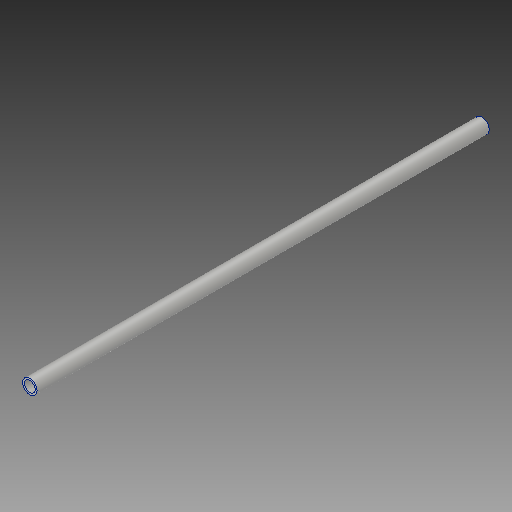
# Autodesk Inventor part: aluminium_bar_D8_L250
Saved by Autodesk Inventor 2019 (Build 230136000, 136)
## iProperties
Created: 2018-10-30
Part Number: aluminium_bar_D8_L250
Material: Aluminum 6061
Document SubType Name: Modeling
Designer: Gianpietro
Density: 2.7 g/cm^3
Appearance: Aluminum - Flat
Mass: 14.844 g
Surface Area: 110.396 cm^2
Volume: 5.49779 cm^3
Author: Gianpietro
Autodesk Inventor part; units mm, degrees
ref_plane "YZ Plane" through (0, 0, 0) normal (1, 0, 0) x (0, 1, 0)
ref_plane "XZ Plane" through (0, 0, 0) normal (0, 1, 0) x (-1, 0, 0)
ref_plane "XY Plane" through (0, 0, 0) normal (0, 0, 1) x (1, 0, 0)
sketch "Sketch1" plane through (0, 0, 0) normal (0, 0, 1) x (1, 0, 0)
  circle A0 centre (0, 0) radius 4
  circle A1 centre (0, 0) radius 3
  dimension "d0" = 8
  dimension "d1" = 6
  constraints: 2 centre point, 2 coincident
  measures "d0" diameter of A0
  measures "d1" diameter of A1
extrude "Extrusion1" add sketch "Sketch1" along normal blind 250
equation "\"d2\" = length"
equation "\"length\" = 250"
body "Solid1"
